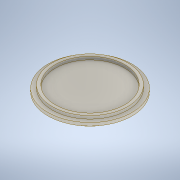
# Autodesk Inventor part: внутреннее кольцо подшипника
Saved by Autodesk Inventor 2020.1 (Build 241239000, 239)
## iProperties
Created: 2022-04-01
Part Number: внутреннее кольцо подшипника
Material: Титан
Document SubType Name: Modeling
Designer: User
Density: 4.51 g/cm^3
Appearance: Титан
Author: User
Autodesk Inventor part; units mm, degrees
ref_plane "YZ Plane" through (0, 0, 0) normal (1, 0, 0) x (0, 1, 0)
ref_plane "XZ Plane" through (0, 0, 0) normal (0, 1, 0) x (-1, 0, 0)
ref_plane "XY Plane" through (0, 0, 0) normal (0, 0, 1) x (1, 0, 0)
sketch "Эскиз1" plane through (0, 0, 0) normal (0, 1, 0) x (-1, 0, 0)
  circle A0 centre (0, 0) radius 55
  dimension "d0" = 110
  constraints: 1 centre point, 1 coincident
  measures "d0" diameter of A0
extrude "Выдавливание1" add sketch "Эскиз1" along normal mid plane 4
sketch "Эскиз2" plane through (0, 0, 0) normal (0, 1, 0) x (-1, 0, 0)
  circle A0 centre (0, 0) radius 55 projected
  circle A1 centre (0, 0) radius 49.5
  circle A2 centre (0, 0) radius 45.5
  point P0 (0, 49.5)
  point P1 (0, 45.5)
  dimension "d4" = 99
  dimension "d5" = 4
  constraints: 2 coincident, 2 vertical alignment, 4 other
  measures "d5" distance of point (0, 45.5) point (0, 49.5)
extrude "Выдавливание2" add sketch "Эскиз2" along normal mid plane 12 contours A1
